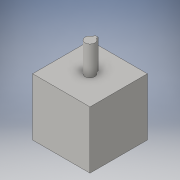
# Autodesk Inventor part: MainMotor
Saved by Autodesk Inventor 2016 (Build 200138000, 138)
## iProperties
Created: 2015-11-30
Part Number: MainMotor
Material: Generic
Document SubType Name: Modeling
Designer: Javier
Density: 1 g/cm^3
Appearance: Default
Author: Javier
Autodesk Inventor part; units mm, degrees
ref_plane "YZ Plane" through (0, 0, 0) normal (1, 0, 0) x (0, 1, 0)
ref_plane "XY Plane" through (0, 0, 0) normal (0, 0, 1) x (1, 0, 0)
sketch "Sketch1" plane through (0, 0, 0) normal (0, 1, 0) x (-1, 0, 0)
  line L0 (49.5033, -49.5033) -> (-60.5041, -49.5033)
  line L1 (-60.5041, -49.5033) -> (-60.5041, 60.5041)
  line L2 (-60.5041, 60.5041) -> (49.5033, 60.5041)
  line L3 (49.5033, 60.5041) -> (49.5033, -49.5033)
  point P0 (0, 0)
  dimension "d0" = 110.0074
  constraints: 8 end point, 2 parallel, 2 perpendicular, 1 horizontal
  measures "d0" distance of L0.end L0.start
extrude "Extrusion1" add sketch "Sketch1" along normal blind 110.0074
ref_plane "Work Plane1" through (0, 110.0074, 0) normal (0, 1, 0) x (-1, 0, 0)
sketch "Sketch2" plane through (0, 110.0074, 0) normal (0, 1, 0) x (-1, 0, 0)
  circle A0 centre (-5.5004, 5.5977) radius 9.4996
  line L0 (-60.5041, 60.5041) -> (-60.5041, -49.5033) projected
  line L1 (49.5033, -49.5033) -> (49.5033, 60.5041) projected
  line L2 (-2.3762, -7.0261) -> (-8.6246, -7.0261)
  line L3 (-8.6246, -7.0261) -> (-8.6246, -3.3735)
  line L4 (-2.3762, -7.0261) -> (-2.3762, -3.3735)
  point P0 (0, 0)
  dimension "d4" = 18.9992
  dimension "d5" = 55.0037
  dimension "d8" = 6.2484
  dimension "d9" = 3.1242
  constraints: 6 end point, 2 point on circle, 1 centre point, 1 perpendicular, 1 vertical
  measures "d4" diameter of A0
  measures "d5" distance from line of L0 A0.centre
  measures "d8" distance of L2.end L2.start
  measures "d9" distance edge to line of A0 L2
extrude "Extrusion2" add sketch "Sketch2" along normal blind 56.007
body "Solid1"
